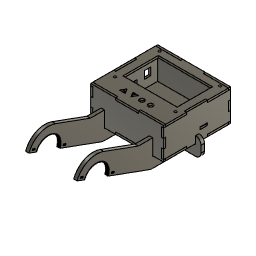
console (Autodesk Fusion 360 design; units mm, degrees)
Autodesk Fusion 360 part; units mm, degrees
sketch "Sketch2" plane through (0, 0, 0) normal (0, 0, 1) x (1, 0, 0)
  line L0 (-39.35, 25.65) -> (39.35, 25.65)
  line L1 (39.35, 25.65) -> (39.35, -25.65)
  line L2 (39.35, -25.65) -> (-39.35, -25.65)
  line L3 (-39.35, -25.65) -> (-39.35, 25.65)
  line L4 (-39.35, 25.65) -> (39.35, -25.65) construction
  line L5 (49.65, 35.65) -> (-50.35, 35.65)
  line L6 (-50.35, 35.65) -> (-50.35, -55.65)
  line L7 (-50.35, -55.65) -> (49.65, -55.65)
  line L8 (49.65, -55.65) -> (49.65, 35.65)
  line L9 (0, 35.516) -> (0, -32.6985) construction
  line L10 (-53.35, -58.65) -> (52.65, -58.65)
  line L11 (52.65, -58.65) -> (52.65, 38.65)
  line L12 (52.65, 38.65) -> (-53.35, 38.65)
  line L13 (-53.35, 38.65) -> (-53.35, -58.65)
  line L14 (-50.35, -55.65) -> (-53.35, -55.65)
  line L15 (-53.35, -25.2167) -> (-50.35, -25.2167)
  line L16 (-50.35, 5.2167) -> (-53.35, 5.2167)
  line L17 (-50.35, 35.65) -> (-53.35, 35.65)
  line L18 (-50.35, 35.65) -> (-50.35, 38.65)
  line L19 (-17.0167, 35.65) -> (-17.0167, 38.65)
  line L20 (16.3167, 35.65) -> (16.3167, 38.65)
  line L21 (49.65, 35.65) -> (49.65, 38.65)
  line L22 (49.65, 35.65) -> (52.65, 35.65)
  line L23 (49.65, 5.2167) -> (52.65, 5.2167)
  line L24 (49.65, -55.65) -> (52.65, -55.65)
  line L25 (49.65, -55.65) -> (49.65, -58.65)
  line L26 (16.3167, -55.65) -> (16.3167, -58.65)
  line L27 (-17.0167, -55.65) -> (-17.0167, -58.65)
  line L28 (-50.35, -55.65) -> (-50.35, -58.65)
  line L29 (-50.35, 37.15) -> (-17.0167, 37.15) construction
  line L30 (-17.0167, 37.15) -> (16.3167, 37.15) construction
  line L31 (16.3167, 37.15) -> (49.65, 37.15) construction
  line L32 (-51.85, 35.65) -> (-51.85, 5.2167) construction
  line L33 (-51.85, 5.2167) -> (-51.85, -25.2167) construction
  line L34 (-51.85, -25.2167) -> (-51.85, -55.65) construction
  line L35 (-50.35, -57.15) -> (-17.0167, -57.15) construction
  line L36 (-17.0167, -57.15) -> (16.3167, -57.15) construction
  line L37 (16.3167, -57.15) -> (49.65, -57.15) construction
  line L38 (49.65, -25.2167) -> (52.65, -25.2167)
  line L39 (51.15, -55.65) -> (51.15, -25.2167) construction
  line L40 (51.15, -25.2167) -> (51.15, 5.2167) construction
  line L41 (51.15, 5.2167) -> (51.15, 35.65) construction
  dimension "d1" = 78.7
  dimension "d2" = 51.3
  dimension "d3" = 100
  dimension "d4" = 10
  dimension "d6" = 30
  dimension "d16" = 3
  dimension "d113" = 11
  constraint horizontal L0
  constraint vertical L1
  constraint horizontal L2
  constraint vertical L3
  constraint midpoint origin L4
  constraint horizontal L5
  constraint vertical L6
  constraint horizontal L7
  constraint vertical L8
  constraint coincident origin L9
  constraint vertical L9
  constraint coincident L13 L14.end
  constraint perpendicular L13 L14
  constraint coincident L13 L15.start
  constraint coincident L6 L15.end
  constraint perpendicular L6 L15
  constraint coincident L6 L16.start
  constraint coincident L13 L16.end
  constraint perpendicular L13 L16
  constraint coincident L13 L17.end
  constraint perpendicular L13 L17
  constraint coincident L12 L18.end
  constraint perpendicular L12 L18
  constraint coincident L5 L19.start
  constraint coincident L12 L19.end
  constraint perpendicular L12 L19
  constraint coincident L5 L20.start
  constraint coincident L12 L20.end
  constraint perpendicular L12 L20
  constraint coincident L12 L21.end
  constraint perpendicular L12 L21
  constraint coincident L11 L22.end
  constraint perpendicular L11 L22
  constraint coincident L8 L23.start
  constraint coincident L11 L23.end
  constraint perpendicular L11 L23
  constraint coincident L11 L24.end
  constraint perpendicular L11 L24
  constraint coincident L10 L25.end
  constraint perpendicular L10 L25
  constraint coincident L7 L26.start
  constraint coincident L10 L26.end
  constraint perpendicular L10 L26
  constraint coincident L7 L27.start
  constraint coincident L10 L27.end
  constraint perpendicular L10 L27
  constraint coincident L10 L28.end
  constraint perpendicular L10 L28
  constraint midpoint L18 L29.start
  constraint midpoint L19 L29.end
  constraint midpoint L20 L30.end
  constraint midpoint L21 L31.end
  constraint equal L30 L31
  constraint equal L29 L30
  constraint midpoint L17 L32.start
  constraint midpoint L16 L32.end
  constraint midpoint L15 L33.end
  constraint midpoint L14 L34.end
  constraint equal L33 L34
  constraint equal L32 L34
  constraint midpoint L28 L35.start
  constraint midpoint L27 L35.end
  constraint midpoint L26 L36.end
  constraint midpoint L25 L37.end
  constraint equal L36 L37
  constraint equal L35 L36
  constraint coincident L8 L38.start
  constraint coincident L11 L38.end
  constraint perpendicular L11 L38
  constraint midpoint L24 L39.start
  constraint midpoint L38 L39.end
  constraint midpoint L23 L40.end
  constraint perpendicular L23 L41
  constraint midpoint L22 L41.end
  constraint equal L40 L41
  constraint equal L39 L40
  measures "d1" distance of L0.start L0.end
  measures "d2" distance of L0.end L1.end
  measures "d3" distance of L5.start L5.end
  measures "d4" distance of L0 L5
  measures "d6" distance of L2 L7
  measures "d113" distance of L3 L6
extrude "Extrude1" add sketch "Sketch2" along normal blind 3 contours L5 L6 L7 L8 | L8 L11 L22 L23 | L5 L12 L19 L20 | L8 L11 L24 L38 | L6 L13 L16 L17 | L7 L10 L26 L27 | L6 L13 L14 L15 makes body 1
sketch "Sketch3" plane through (0, 0, 0) normal (0, 0, -1) x (1, 0, 0)
  line L0 (-39.35, 25.65) -> (39.35, 25.65)
  line L1 (39.35, 25.65) -> (39.35, -25.65)
  line L2 (39.35, -25.65) -> (-39.35, -25.65)
  line L3 (-39.35, -25.65) -> (-39.35, 25.65)
  line L4 (-43.9, 32.65) -> (43.9, 32.65) construction
  line L5 (43.9, 32.65) -> (43.9, -32.15) construction
  line L6 (43.9, -32.15) -> (-43.9, -32.15) construction
  line L7 (-43.9, -32.15) -> (-43.9, 32.65) construction
  line L8 (-43.9, 32.65) -> (43.9, -32.15) construction
  circle A0 centre (-43.9, -32.15) radius 4
  circle A1 centre (43.9, -32.15) radius 4
  circle A2 centre (43.9, 32.65) radius 4
  circle A3 centre (-43.9, 32.65) radius 4
  circle A4 centre (-43.9, 32.65) radius 1.75
  circle A5 centre (43.9, 32.65) radius 1.75
  circle A6 centre (43.9, -32.15) radius 1.75
  circle A7 centre (-43.9, -32.15) radius 1.75
  line L9 (-53.35, 55.65) -> (-53.35, 25.2167)
  line L10 (-17.0167, -38.65) -> (16.3167, -38.65)
  line L11 (52.65, 25.2167) -> (52.65, 55.65)
  line L12 (16.3167, 58.65) -> (-17.0167, 58.65)
  line L13 (52.65, -5.2167) -> (49.65, -5.2167)
  line L14 (49.65, -5.2167) -> (49.65, 25.2167)
  line L15 (49.65, 25.2167) -> (52.65, 25.2167)
  line L16 (52.65, 55.65) -> (16.3167, 55.65)
  line L17 (16.3167, 55.65) -> (16.3167, 58.65)
  line L18 (-17.0167, 58.65) -> (-17.0167, 55.65)
  line L19 (-17.0167, 55.65) -> (-53.35, 55.65)
  line L20 (-53.35, 25.2167) -> (-50.35, 25.2167)
  line L21 (-50.35, 25.2167) -> (-50.35, -5.2167)
  line L22 (-50.35, -5.2167) -> (-53.35, -5.2167)
  line L23 (-53.35, -5.2167) -> (-53.35, -35.65)
  line L24 (-53.35, -35.65) -> (-17.0167, -35.65)
  line L25 (-17.0167, -35.65) -> (-17.0167, -38.65)
  line L26 (16.3167, -38.65) -> (16.3167, -35.65)
  line L27 (16.3167, -35.65) -> (52.65, -35.65)
  line L28 (52.65, -35.65) -> (52.65, -5.2167)
  line L29 (49.65, 55.65) -> (49.65, -35.65)
  line L30 (-17.0167, -35.65) -> (-53.35, -35.65)
  line L31 (0, 0) -> (0, 0.25) construction
  dimension "d9" = 87.8
  dimension "d10" = 64.8
  dimension "d11" = 8
  dimension "d12" = 3.5
  dimension "d55" = 3.5
  constraint horizontal L4
  constraint vertical L5
  constraint horizontal L6
  constraint vertical L7
  constraint coincident L6.end L7.start
  constraint coincident L5.end L6.start
  constraint coincident L4.end L5.start
  constraint coincident L4.start L7.end
  constraint equal A2 A3
  constraint equal A0 A3
  constraint equal A0 A1
  constraint concentric A3 A4
  constraint concentric A2 A5
  constraint concentric A1 A6
  constraint equal A6 A7
  constraint equal A4 A7
  constraint equal A4 A5
  constraint coincident L16 L29.start
  constraint coincident L27 L29.end
  constraint vertical L29
  constraint collinear L14 L29
  constraint coincident L31.start origin
  constraint midpoint L8 L31.end
  constraint vertical L31
  measures "d9" distance of L4.start L4.end
  measures "d10" distance of L4.end L5.end
  measures "d11" diameter of A1
  measures "d12" diameter of A4
  measures "d55" distance of L6 L30
extrude "Extrude2" add sketch "Sketch3" along normal blind 3 separate body contours A0 L24 L30 | A1 L27 | A2 | A3 picked at (-43.8564, -35.065) picked at (43.4291, -35.7307) makes body 2 at (47.895, -32.4506, -2) makes body 3 at (45.6659, 35.7391, -2) makes body 4 at (-39.905, -32.4506, -2) makes body 5 at (-42.3772, 28.4512, -1)
sketch "Sketch5" plane through (-50.35, 0, 0) normal (-1, 0, 0) x (0, -1, 0)
  line L0 (-5.2167, 0) -> (25.2167, 0)
  line L1 (25.2167, 0) -> (25.2167, 3)
  line L2 (25.2167, 3) -> (-5.2167, 3)
  line L3 (-5.2167, 3) -> (-5.2167, 0)
  line L4 (-38.65, 0) -> (-35.65, 0)
  line L5 (-35.65, 0) -> (-35.65, 3)
  line L6 (-35.65, 3) -> (-38.65, 3)
  line L7 (-38.65, 3) -> (-38.65, 0)
  line L8 (-35.65, 0) -> (-5.2167, 0)
  line L9 (-5.2167, 0) -> (-5.2167, 3)
  line L10 (-5.2167, 3) -> (-35.65, 3)
  line L11 (-35.65, 3) -> (-35.65, 0)
  line L12 (25.2167, 0) -> (55.65, 0)
  line L13 (55.65, 0) -> (55.65, 3)
  line L14 (55.65, 3) -> (25.2167, 3)
  line L15 (25.2167, 3) -> (25.2167, 0)
  line L16 (55.65, 0) -> (58.65, 0)
  line L17 (58.65, 0) -> (58.65, 3)
  line L18 (58.65, 3) -> (55.65, 3)
  line L19 (55.65, 3) -> (55.65, 0)
  line L20 (-35.65, 0) -> (55.65, 0)
  line L21 (55.65, 0) -> (55.65, -40)
  line L22 (55.65, -40) -> (-35.65, -40)
  line L23 (-35.65, -40) -> (-35.65, 0)
  line L24 (25.2167, 0) -> (55.65, 0)
  line L25 (-38.65, 0) -> (-35.65, 0)
  line L26 (-35.65, 0) -> (-35.65, -13.3333)
  line L27 (-35.65, -13.3333) -> (-38.65, -13.3333)
  line L28 (-38.65, -13.3333) -> (-38.65, 0)
  line L29 (-35.65, -40) -> (-38.65, -40)
  line L30 (-38.65, -40) -> (-38.65, -26.6667)
  line L31 (-38.65, -26.6667) -> (-35.65, -26.6667)
  line L32 (-35.65, -26.6667) -> (-35.65, -40)
  line L33 (-38.65, -13.3333) -> (-38.65, -26.6667) construction
  line L34 (55.65, 0) -> (58.65, 0)
  line L35 (58.65, 0) -> (58.65, -13.3333)
  line L36 (58.65, -13.3333) -> (55.65, -13.3333)
  line L37 (55.65, -13.3333) -> (55.65, 0)
  line L38 (55.65, -40) -> (58.65, -40)
  line L39 (58.65, -40) -> (58.65, -26.6667)
  line L40 (58.65, -26.6667) -> (55.65, -26.6667)
  line L41 (55.65, -26.6667) -> (55.65, -40)
  line L42 (58.65, -13.3333) -> (58.65, -26.6667) construction
  line L43 (-5.2167, -40) -> (25.2167, -40)
  line L44 (25.2167, -40) -> (25.2167, -43)
  line L45 (25.2167, -43) -> (-5.2167, -43)
  line L46 (-5.2167, -43) -> (-5.2167, -40)
  dimension "d31" = 40
  constraint horizontal L20
  constraint vertical L21
  constraint horizontal L22
  constraint vertical L23
  constraint coincident L4.end L5.start
  constraint coincident L12.end L13.start
  constraint horizontal L25
  constraint vertical L26
  constraint horizontal L27
  constraint vertical L28
  constraint coincident L23 L26.end
  constraint coincident L4.start L7.end
  constraint horizontal L29
  constraint vertical L30
  constraint horizontal L31
  constraint vertical L32
  constraint perpendicular L31 L33
  constraint equal L28 L33
  constraint equal L28 L30
  constraint horizontal L34
  constraint vertical L35
  constraint horizontal L36
  constraint vertical L37
  constraint coincident L16.end L17.start
  constraint horizontal L38
  constraint vertical L39
  constraint horizontal L40
  constraint vertical L41
  constraint collinear L35 L39
  constraint equal L35 L42
  constraint equal L35 L39
  constraint horizontal L43
  constraint vertical L44
  constraint horizontal L45
  constraint vertical L46
  constraint coincident L22 L43.start
  constraint equal L1 L44
  constraint equal L2 L45
  constraint collinear L3 L46
  measures "d31" distance of L22 L24
extrude "Extrude6" add sketch "Sketch5" along normal blind 3 separate body contours L0 L1 L2 L3 L9 L15 L20 | L0 L8 L12 L20 L21 L22 L23 L24 L26 L32 L37 L41 L43 | L4 L23 L25 L26 L27 L28 | L16 L21 L34 L35 L36 L37 | L23 L29 L30 L31 L32 | L21 L38 L39 L40 L41 | L22 L43 L44 L45 L46 makes body 6
sketch "Sketch4" plane through (-53.35, 0, 0) normal (-1, 0, 0) x (0, -1, 0)
  line L0 (25.2167, 0) -> (55.65, 0)
  line L1 (55.65, 0) -> (55.65, 3)
  line L2 (55.65, 3) -> (25.2167, 3)
  line L3 (25.2167, 3) -> (25.2167, 0)
  line L4 (-35.65, 0) -> (-5.2167, 0)
  line L5 (-5.2167, 0) -> (-5.2167, 3)
  line L6 (-5.2167, 3) -> (-35.65, 3)
  line L7 (-35.65, 3) -> (-35.65, 0)
  line L8 (-25.65, -17) -> (-16.65, -17)
  line L9 (-16.65, -17) -> (-16.65, -28)
  line L10 (-16.65, -28) -> (-25.65, -28)
  line L11 (-25.65, -28) -> (-25.65, -17)
  line L12 (-25.65, 3) -> (-25.65, -17) construction
  line L13 (-5.65, -31) -> (6.35, -31)
  line L14 (6.35, -31) -> (6.35, -23)
  line L15 (6.35, -23) -> (-5.65, -23)
  line L16 (-5.65, -23) -> (-5.65, -31)
  line L17 (-5.65, -23) -> (6.35, -31) construction
  point P0 (-25.65, 3)
  point P1 (25.65, 3)
  point P2 (0.35, -27)
  dimension "d114" = 17
  dimension "d115" = 11
  dimension "d116" = 9
  dimension "d118" = 17
  dimension "d119" = 12
  dimension "d120" = 8
  dimension "d125" = 1
  constraint horizontal L8
  constraint vertical L9
  constraint horizontal L10
  constraint vertical L11
  constraint coincident P0 L12.start
  constraint vertical L12
  constraint horizontal L13
  constraint vertical L14
  constraint horizontal L15
  constraint vertical L16
  constraint midpoint L17 P2
  measures "d114" distance of L4 L8
  measures "d115" distance of L8.end L9.end
  measures "d116" distance of L9.end L10.end
  measures "d118" distance of L9 P2
  measures "d119" distance of L14.end L15.end
  measures "d120" distance of L13.end L14.end
  measures "d125" distance of L10 P2
extrude "Extrude7" cut sketch "Sketch4" against normal through all contours L8 L9 L10 L11 | L13 L14 L15 L16 bodies 6
extrude "Extrude8" cut sketch "Sketch3" against normal through all contours A4 | A5 | A6 | A7 bodies 1
sketch "Sketch6" plane through (49.65, 0, 0) normal (1, 0, 0) x (0, 1, 0)
  line L0 (-58.65, -40) -> (-25.2167, -40)
  line L1 (-25.2167, -40) -> (-25.2167, -43)
  line L2 (-25.2167, -43) -> (5.2167, -43)
  line L3 (5.2167, -43) -> (5.2167, -40)
  line L4 (5.2167, -40) -> (38.65, -40)
  line L5 (38.65, -40) -> (38.65, -26.6667)
  line L6 (38.65, -26.6667) -> (35.65, -26.6667)
  line L7 (35.65, -26.6667) -> (35.65, -13.3333)
  line L8 (35.65, -13.3333) -> (38.65, -13.3333)
  line L9 (38.65, -13.3333) -> (38.65, 0)
  line L10 (38.65, 0) -> (5.2167, 0)
  line L11 (5.2167, 0) -> (5.2167, 3)
  line L12 (5.2167, 3) -> (-25.2167, 3)
  line L13 (-25.2167, 3) -> (-25.2167, 0)
  line L14 (-25.2167, 0) -> (-58.65, 0)
  line L15 (-58.65, 0) -> (-58.65, -13.3333)
  line L16 (-58.65, -13.3333) -> (-55.65, -13.3333)
  line L17 (-55.65, -13.3333) -> (-55.65, -26.6667)
  line L18 (-55.65, -26.6667) -> (-58.65, -26.6667)
  line L19 (-58.65, -26.6667) -> (-58.65, -40)
  line L20 (-6.35, -23) -> (5.65, -23)
  line L21 (5.65, -23) -> (5.65, -31)
  line L22 (5.65, -31) -> (-6.35, -31)
  line L23 (-6.35, -31) -> (-6.35, -23)
  line L24 (25.65, -17) -> (25.65, -28)
  line L25 (25.65, -28) -> (16.65, -28)
  line L26 (16.65, -28) -> (16.65, -17)
  line L27 (16.65, -17) -> (25.65, -17)
extrude "Extrude9" add sketch "Sketch6" along normal blind 3 separate body contours L0 L1 L2 L3 L4 L5 L6 L7 L8 L9 L10 L11 L12 L13 L14 L15 L16 L17 L18 L19 | L20 L21 L22 L23 | L24 L25 L26 L27 makes body 7
sketch "Sketch7" plane through (52.65, 0, 0) normal (1, 0, 0) x (0, 1, 0)
  line L0 (-58.65, -26.6667) -> (-58.65, -40)
  line L1 (-58.65, -40) -> (-25.2167, -40)
  line L2 (-25.2167, -40) -> (-25.2167, -43)
  line L3 (-25.2167, -43) -> (5.2167, -43)
  line L4 (5.2167, -43) -> (5.2167, -40)
  line L5 (5.2167, -40) -> (38.65, -40)
  line L6 (38.65, -40) -> (38.65, -26.6667)
  line L7 (38.65, -26.6667) -> (35.65, -26.6667)
  line L8 (35.65, -26.6667) -> (35.65, -13.3333)
  line L9 (35.65, -13.3333) -> (38.65, -13.3333)
  line L10 (38.65, -13.3333) -> (38.65, 0)
  line L11 (38.65, 0) -> (5.2167, 0)
  line L12 (5.2167, 0) -> (5.2167, 3)
  line L13 (5.2167, 3) -> (-25.2167, 3)
  line L14 (-25.2167, 3) -> (-25.2167, 0)
  line L15 (-25.2167, 0) -> (-58.65, 0)
  line L16 (-58.65, 0) -> (-58.65, -13.3333)
  line L17 (-58.65, -13.3333) -> (-55.65, -13.3333)
  line L18 (-55.65, -13.3333) -> (-55.65, -26.6667)
  line L19 (-55.65, -26.6667) -> (-58.65, -26.6667)
  line L20 (-5.6, -25.25) -> (4.9, -25.25)
  line L21 (4.9, -25.25) -> (4.9, -28.75)
  line L22 (4.9, -28.75) -> (-5.6, -28.75)
  line L23 (-5.6, -28.75) -> (-5.6, -25.25)
  line L24 (-6.35, -23) -> (5.65, -23)
  line L25 (5.65, -23) -> (5.65, -31)
  line L26 (5.65, -31) -> (-6.35, -31)
  line L27 (-6.35, -31) -> (-6.35, -23)
  line L28 (-5.6, -25.25) -> (4.9, -28.75) construction
  line L29 (5.65, -31) -> (-6.35, -23) construction
  dimension "d122" = 10.5
  dimension "d123" = 3.5
  constraint horizontal L20
  constraint vertical L21
  constraint horizontal L22
  constraint vertical L23
  constraint coincident L25.end L26.start
  constraint coincident L24.start L27.end
  constraint midpoint L28 L29
  measures "d122" distance of L20.start L20.end
  measures "d123" distance of L20.end L21.end
extrude "Extrude10" cut sketch "Sketch7" against normal through all contours L20 L21 L22 L23 bodies 7
sketch "Sketch8" plane through (0, -55.65, 0) normal (0, -1, 0) x (1, 0, 0)
  line L0 (-53.35, 0) -> (-17.0167, 0)
  line L1 (-17.0167, 0) -> (-17.0167, 3)
  line L2 (-17.0167, 3) -> (-53.35, 3)
  line L3 (-53.35, 3) -> (-53.35, 0)
  line L4 (-17.0167, 0) -> (16.3167, 0)
  line L5 (16.3167, 0) -> (16.3167, 3)
  line L6 (16.3167, 3) -> (-17.0167, 3)
  line L7 (-17.0167, 3) -> (-17.0167, 0)
  line L8 (16.3167, 0) -> (52.65, 0)
  line L9 (52.65, 0) -> (52.65, 3)
  line L10 (52.65, 3) -> (16.3167, 3)
  line L11 (16.3167, 3) -> (16.3167, 0)
  line L12 (49.65, 0) -> (49.65, -13.3333)
  line L13 (49.65, -13.3333) -> (52.65, -13.3333)
  line L14 (52.65, -13.3333) -> (52.65, 0)
  line L15 (52.65, 0) -> (49.65, 0)
  line L16 (49.65, -13.3333) -> (49.65, -26.6667)
  line L17 (49.65, -26.6667) -> (52.65, -26.6667)
  line L18 (52.65, -26.6667) -> (52.65, -13.3333)
  line L19 (52.65, -13.3333) -> (49.65, -13.3333)
  line L20 (49.65, -26.6667) -> (49.65, -40)
  line L21 (49.65, -40) -> (52.65, -40)
  line L22 (52.65, -40) -> (52.65, -26.6667)
  line L23 (52.65, -26.6667) -> (49.65, -26.6667)
  line L24 (-50.35, -40) -> (-50.35, -26.6667)
  line L25 (-50.35, -26.6667) -> (-53.35, -26.6667)
  line L26 (-53.35, -26.6667) -> (-53.35, -40)
  line L27 (-53.35, -40) -> (-50.35, -40)
  line L28 (-50.35, -13.3333) -> (-50.35, 0)
  line L29 (-50.35, 0) -> (-53.35, 0)
  line L30 (-53.35, 0) -> (-53.35, -13.3333)
  line L31 (-53.35, -13.3333) -> (-50.35, -13.3333)
  line L32 (-50.35, -26.6667) -> (-50.35, -13.3333)
  line L33 (-50.35, -13.3333) -> (-53.35, -13.3333)
  line L34 (-53.35, -13.3333) -> (-53.35, -26.6667)
  line L35 (-53.35, -26.6667) -> (-50.35, -26.6667)
  line L36 (-50.35, -40) -> (49.65, -40)
  line L37 (-53.35, -40) -> (-17.0167, -40)
  line L38 (-17.0167, -40) -> (-17.0167, -43)
  line L39 (-17.0167, -43) -> (-53.35, -43)
  line L40 (-53.35, -43) -> (-53.35, -40)
  line L41 (-17.0167, -43) -> (16.3167, -43)
  line L42 (16.3167, -43) -> (16.3167, -40)
  line L43 (16.3167, -40) -> (-17.0167, -40)
  line L44 (-17.0167, -40) -> (-17.0167, -43)
  line L45 (16.3167, -43) -> (52.65, -43)
  line L46 (52.65, -43) -> (52.65, -40)
  line L47 (52.65, -40) -> (16.3167, -40)
  line L48 (16.3167, -40) -> (16.3167, -43)
  constraint coincident L24.start L27.end
  constraint coincident L20.end L21.start
  constraint horizontal L37
  constraint vertical L38
  constraint horizontal L39
  constraint vertical L40
  constraint coincident L26.end L27.start
  constraint horizontal L41
  constraint vertical L42
  constraint horizontal L43
  constraint vertical L44
  constraint coincident L36 L42.end
  constraint horizontal L45
  constraint vertical L46
  constraint horizontal L47
  constraint vertical L48
  constraint coincident L21.end L22.start
  constraint collinear L11 L48
  constraint collinear L1 L38
  constraint equal L1 L38
extrude "Extrude11" add sketch "Sketch8" along normal blind 3 separate body contours L0 L1 L2 L3 L7 L29 | L0 L4 L8 L12 L16 L20 L24 L28 L32 L36 L37 L43 L47 | L25 L31 L32 L33 L34 L35 | L5 L8 L9 L10 L11 L15 | L27 L36 L37 L38 L39 L40 L44 | L13 L16 L17 L18 L19 L23 | L21 L36 L42 L45 L46 L47 L48 makes body 8
sketch "Sketch9" plane through (0, 35.65, 0) normal (0, 1, 0) x (-1, 0, 0)
  line L0 (-52.65, 0) -> (-16.3167, 0)
  line L1 (-16.3167, 0) -> (-16.3167, 3)
  line L2 (-16.3167, 3) -> (-52.65, 3)
  line L3 (-52.65, 3) -> (-52.65, 0)
  line L4 (-16.3167, -40) -> (17.0167, -40)
  line L5 (17.0167, -40) -> (17.0167, -43)
  line L6 (17.0167, -43) -> (53.35, -43)
  line L7 (53.35, -43) -> (53.35, -40)
  line L8 (53.35, -40) -> (50.35, -40)
  line L9 (50.35, -40) -> (50.35, -26.6667)
  line L10 (50.35, -26.6667) -> (53.35, -26.6667)
  line L11 (53.35, -26.6667) -> (53.35, -13.3333)
  line L12 (53.35, -13.3333) -> (50.35, -13.3333)
  line L13 (50.35, -13.3333) -> (50.35, 0)
  line L14 (50.35, 0) -> (53.35, 0)
  line L15 (53.35, 0) -> (53.35, 3)
  line L16 (53.35, 3) -> (17.0167, 3)
  line L17 (17.0167, 3) -> (17.0167, 0)
  line L18 (17.0167, 0) -> (-16.3167, 0)
  line L19 (-16.3167, 0) -> (-16.3167, 3)
  line L20 (-16.3167, 3) -> (-52.65, 3)
  line L21 (-52.65, 3) -> (-52.65, 0)
  line L22 (-52.65, 0) -> (-49.65, 0)
  line L23 (-49.65, 0) -> (-49.65, -13.3333)
  line L24 (-49.65, -13.3333) -> (-52.65, -13.3333)
  line L25 (-52.65, -13.3333) -> (-52.65, -26.6667)
  line L26 (-52.65, -26.6667) -> (-49.65, -26.6667)
  line L27 (-49.65, -26.6667) -> (-49.65, -40)
  line L28 (-49.65, -40) -> (-52.65, -40)
  line L29 (-52.65, -40) -> (-52.65, -43)
  line L30 (-52.65, -43) -> (-16.3167, -43)
  line L31 (-16.3167, -43) -> (-16.3167, -40)
extrude "Extrude12" add sketch "Sketch9" along normal blind 3 separate body makes body 9
sketch "Sketch10" plane through (0, 0, -40) normal (0, 0, -1) x (1, 0, 0)
  line L0 (52.65, -5.2167) -> (49.65, -5.2167)
  line L1 (49.65, -5.2167) -> (49.65, 25.2167)
  line L2 (49.65, 25.2167) -> (52.65, 25.2167)
  line L3 (52.65, 25.2167) -> (52.65, 55.65)
  line L4 (52.65, 55.65) -> (16.3167, 55.65)
  line L5 (16.3167, 55.65) -> (16.3167, 58.65)
  line L6 (16.3167, 58.65) -> (-17.0167, 58.65)
  line L7 (-17.0167, 58.65) -> (-17.0167, 55.65)
  line L8 (-17.0167, 55.65) -> (-53.35, 55.65)
  line L9 (-53.35, 55.65) -> (-53.35, 25.2167)
  line L10 (-53.35, 25.2167) -> (-50.35, 25.2167)
  line L11 (-50.35, 25.2167) -> (-50.35, -5.2167)
  line L12 (-50.35, -5.2167) -> (-53.35, -5.2167)
  line L13 (-53.35, -5.2167) -> (-53.35, -35.65)
  line L14 (-53.35, -35.65) -> (-17.0167, -35.65)
  line L15 (-17.0167, -35.65) -> (-17.0167, -38.65)
  line L16 (-17.0167, -38.65) -> (16.3167, -38.65)
  line L17 (16.3167, -38.65) -> (16.3167, -35.65)
  line L18 (16.3167, -35.65) -> (52.65, -35.65)
  line L19 (52.65, -35.65) -> (52.65, -5.2167)
extrude "Extrude13" add sketch "Sketch10" along normal blind 3 separate body makes body 10
sketch "Sketch11" plane through (0, 0, 3) normal (0, 0, 1) x (-1, 0, 0)
  circle A0 centre (-43.9, 32.65) radius 1.75
  circle A1 centre (-43.9, -32.15) radius 1.75
  circle A2 centre (43.9, 32.65) radius 1.75
  circle A3 centre (43.9, -32.15) radius 1.75
  line L0 (-39.35, 25.65) -> (39.35, 25.65)
  line L1 (39.35, 25.65) -> (39.35, -25.65)
  line L2 (39.35, -25.65) -> (-39.35, -25.65)
  line L3 (-39.35, -25.65) -> (-39.35, 25.65)
  line L4 (-49.65, -5.2167) -> (-52.65, -5.2167)
  line L5 (-52.65, -5.2167) -> (-52.65, -35.65)
  line L6 (-52.65, -35.65) -> (-16.3167, -35.65)
  line L7 (-16.3167, -35.65) -> (-16.3167, -38.65)
  line L8 (-16.3167, -38.65) -> (17.0167, -38.65)
  line L9 (17.0167, -38.65) -> (17.0167, -35.65)
  line L10 (17.0167, -35.65) -> (53.35, -35.65)
  line L11 (53.35, -35.65) -> (53.35, -5.2167)
  line L12 (53.35, -5.2167) -> (50.35, -5.2167)
  line L13 (50.35, -5.2167) -> (50.35, 25.2167)
  line L14 (50.35, 25.2167) -> (53.35, 25.2167)
  line L15 (53.35, 25.2167) -> (53.35, 55.65)
  line L16 (53.35, 55.65) -> (17.0167, 55.65)
  line L17 (17.0167, 55.65) -> (17.0167, 58.65)
  line L18 (17.0167, 58.65) -> (-16.3167, 58.65)
  line L19 (-16.3167, 58.65) -> (-16.3167, 55.65)
  line L20 (-16.3167, 55.65) -> (-52.65, 55.65)
  line L21 (-52.65, 55.65) -> (-52.65, 25.2167)
  line L22 (-52.65, 25.2167) -> (-49.65, 25.2167)
  line L23 (-49.65, 25.2167) -> (-49.65, -5.2167)
  line L24 (50.35, 25.2167) -> (50.35, 55.65)
  line L25 (50.35, 35.65) -> (-48.1566, 35.65)
  line L26 (-49.65, 25.2167) -> (-49.65, 55.65)
  line L27 (19.8467, 42.65) -> (7.3467, 42.65) construction
  line L28 (7.3467, 42.65) -> (-5.1533, 42.65) construction
  line L29 (-5.1533, 42.65) -> (-17.6533, 42.65) construction
  line L30 (1.0967, 42.65) -> (1.0967, 35.65) construction
  line L31 (17.0167, 55.65) -> (-16.3167, 55.65) construction
  line L32 (23.8467, 46.1141) -> (15.8467, 46.1141)
  line L33 (15.8467, 46.1141) -> (19.8467, 39.1859)
  line L34 (19.8467, 39.1859) -> (23.8467, 46.1141)
  line L35 (11.3467, 39.1859) -> (3.3467, 39.1859)
  line L36 (3.3467, 39.1859) -> (7.3467, 46.1141)
  line L37 (7.3467, 46.1141) -> (11.3467, 39.1859)
  line L38 (7.3467, 39.1859) -> (7.3467, 46.1141) construction
  line L39 (19.8467, 39.1859) -> (19.8467, 46.1141) construction
  circle A4 centre (-5.1533, 42.65) radius 3.4641
  circle A5 centre (-17.6533, 42.65) radius 3.4641
  point P0 (19.8467, 42.65)
  point P1 (7.3467, 42.65)
  dimension "d50" = 10
  dimension "d51" = 12.5
  dimension "d52" = 8
  dimension "d54" = 7
  constraint coincident L13.end L14.start
  constraint coincident L16 L24.end
  constraint perpendicular L16 L24
  constraint coincident L24 L25.start
  constraint perpendicular L24 L25
  constraint coincident L22.end L23.start
  constraint coincident L20 L26.end
  constraint perpendicular L20 L26
  constraint horizontal L27
  constraint parallel L27 L28
  constraint parallel L28 L29
  constraint equal L28 L29
  constraint equal L27 L28
  constraint midpoint L28 L30.start
  constraint midpoint L25 L30.end
  constraint perpendicular L25 L30
  constraint coincident L16.end L17.start
  constraint coincident L19.end L20.start
  constraint perpendicular L1 L32
  constraint equal L32 L34
  constraint equal L32 L33
  constraint coincident L27 P0
  constraint coincident P0 L27.start
  constraint parallel L27 L35
  constraint equal L35 L37
  constraint equal L35 L36
  constraint equal L33 L37
  constraint midpoint L35 L38.start
  constraint coincident L38 P1
  constraint midpoint L38 P1
  constraint midpoint L32 L39.end
  constraint midpoint P0 L39
  constraint coincident P1 L27.end
  constraint coincident L28.end L29.start
  constraint coincident L29.end A5.centre
  constraint tangent L35 A4
  constraint equal A4 A5
  measures "d50" distance of L0 L25
  measures "d51" distance of P0 P1
  measures "d52" distance of L35.start L35.end
  measures "d54" distance of L30.start L30.end
extrude "Extrude14" cut sketch "Sketch11" against normal through all contours L32 L33 L34 | L35 L36 L37 | A4 | A5 bodies 1
sketch "Sketch14" plane through (0, 0, 3) normal (0, 0, 1) x (-1, 0, 0)
  line L0 (3.3467, 39.1859) -> (7.3467, 46.1141)
  line L1 (7.3467, 46.1141) -> (11.3467, 39.1859)
  line L2 (11.3467, 39.1859) -> (3.3467, 39.1859)
  circle A0 centre (-5.1533, 42.65) radius 3.4641
  line L3 (23.8467, 46.1141) -> (19.8467, 39.1859)
  line L4 (19.8467, 39.1859) -> (15.8467, 46.1141)
  line L5 (15.8467, 46.1141) -> (23.8467, 46.1141)
  circle A1 centre (-17.6533, 42.65) radius 3.4641
  circle A2 centre (-43.9, 32.65) radius 1.75
  circle A3 centre (-43.9, -32.15) radius 1.75
  circle A4 centre (43.9, 32.65) radius 1.75
  circle A5 centre (43.9, -32.15) radius 1.75
  line L6 (-39.35, 25.65) -> (39.35, 25.65)
  line L7 (39.35, 25.65) -> (39.35, -25.65)
  line L8 (39.35, -25.65) -> (-39.35, -25.65)
  line L9 (-39.35, -25.65) -> (-39.35, 25.65)
  line L10 (-49.65, -5.2167) -> (-52.65, -5.2167)
  line L11 (-52.65, -5.2167) -> (-52.65, -35.65)
  line L12 (-52.65, -35.65) -> (-16.3167, -35.65)
  line L13 (-16.3167, -35.65) -> (-16.3167, -38.65)
  line L14 (-16.3167, -38.65) -> (17.0167, -38.65)
  line L15 (17.0167, -38.65) -> (17.0167, -35.65)
  line L16 (17.0167, -35.65) -> (53.35, -35.65)
  line L17 (53.35, -35.65) -> (53.35, -5.2167)
  line L18 (53.35, -5.2167) -> (50.35, -5.2167)
  line L19 (50.35, -5.2167) -> (50.35, 25.2167)
  line L20 (50.35, 25.2167) -> (53.35, 25.2167)
  line L21 (53.35, 25.2167) -> (53.35, 55.65)
  line L22 (53.35, 55.65) -> (17.0167, 55.65)
  line L23 (17.0167, 55.65) -> (17.0167, 58.65)
  line L24 (17.0167, 58.65) -> (-16.3167, 58.65)
  line L25 (-16.3167, 58.65) -> (-16.3167, 55.65)
  line L26 (-16.3167, 55.65) -> (-52.65, 55.65)
  line L27 (-52.65, 55.65) -> (-52.65, 25.2167)
  line L28 (-52.65, 25.2167) -> (-49.65, 25.2167)
  line L29 (-49.65, 25.2167) -> (-49.65, -5.2167)
  circle A6 centre (-17.6533, 42.65) radius 3.1641
  circle A7 centre (-5.1533, 42.65) radius 3.1641
  line L30 (7.3467, 45.5141) -> (10.8271, 39.4859)
  line L31 (10.8271, 39.4859) -> (3.8663, 39.4859)
  line L32 (3.8663, 39.4859) -> (7.3467, 45.5141)
  line L33 (23.3271, 45.8141) -> (19.8467, 39.7859)
  line L34 (19.8467, 39.7859) -> (16.3663, 45.8141)
  line L35 (16.3663, 45.8141) -> (23.3271, 45.8141)
  line L36 (26.4448, 47.6141) -> (19.8467, 36.1859)
  line L37 (19.8467, 36.1859) -> (13.2486, 47.6141)
  line L38 (13.2486, 47.6141) -> (26.4448, 47.6141)
  line L39 (7.3467, 49.1141) -> (13.9448, 37.6859)
  line L40 (13.9448, 37.6859) -> (0.7486, 37.6859)
  line L41 (0.7486, 37.6859) -> (7.3467, 49.1141)
  circle A8 centre (-5.1533, 42.65) radius 4.9641
  circle A9 centre (-17.6533, 42.65) radius 4.9641
  line L42 (29.4429, 46.1141) -> (27.8654, 46.1141)
  line L43 (27.8654, 46.1141) -> (-27.5893, 46.1141)
  dimension "d59" = -0.3
  dimension "d60" = -0.3
  dimension "d61" = 0.3
  dimension "d62" = 0.3
  dimension "d63" = -1.5
  dimension "d64" = -1.5
  dimension "d65" = 1.5
  dimension "d66" = 1.5
  constraint parallel L35 L42
  constraint parallel L42 L43
  constraint collinear L5 L43
extrude "Extrude15" add sketch "Sketch14" against normal blind 4 from surface at 1 separate body contours A6 | A7 | L30 L31 L32 | L33 L34 L35 makes body 11 at (-8.5069, -43.5047, 2.6667) makes body 12 at (2.0049, -42.335, 1.3333) makes body 13 at (-18.6866, -41.7953, 2.6667) makes body 14 at (14.5049, -42.335, 1.3333)
extrude "Extrude16" add sketch "Sketch14" against normal blind 2 from surface at -3 contours L39 L40 L41 L43 | L0 L1 L2 | A0 | A8 L43 | L3 L4 L36 L37 L43 | L3 L4 L5 L43 | A1 | A9 L43 | A6 | A7 | L30 L31 L32 | L33 L34 L35 picked at (-8.5706, 45.5086) picked at (-21.0706, 45.5086) bodies 11 12 13 14
fillet "Fillet2" radius 1 4 faces at (-7.3467, -41.4953, 4) (5.9685, -41.8254, 4) (-19.8467, -43.8047, 4) (19.3399, -43.3348, 4) on bodies 11 12 13 14
ref_plane "WorkPlane3" through (-0.35, -10, -20) normal (1, 0, 0) x (0, 0, -1)
sketch "Sketch15" plane through (-0.35, 0, 0) normal (1, 0, 0) x (0, 1, 0)
  circle A0 centre (-140.6017, -29.7621) radius 17.75
  line L0 (38.5, 0) -> (38.5, -13.3333)
  line L1 (38.5, -26.6667) -> (38.5, -13.3333)
  line L2 (38.5, -26.6667) -> (38.5, -40)
  line L3 (38.5, -43) -> (38.5, -40)
  line L4 (35.5, -43) -> (38.5, -43)
  line L5 (5.1667, -43) -> (35.5, -43)
  line L6 (5.1667, -43) -> (-25.1667, -43)
  line L7 (-55.5, -43) -> (-25.1667, -43)
  line L8 (-55.5, -43) -> (-58.5, -43)
  line L9 (-58.5, -40) -> (-58.5, -43)
  line L10 (-58.5, -40) -> (-58.5, -26.6667)
  line L11 (-58.5, -13.3333) -> (-58.5, -26.6667)
  line L12 (-58.5, -13.3333) -> (-58.5, 0)
  line L13 (39, 0) -> (39, -13.3333)
  line L14 (39, -26.6667) -> (39, -13.3333)
  line L15 (39, -26.6667) -> (39, -40)
  line L16 (39, -43.5) -> (39, -40)
  line L17 (35.5, -43.5) -> (39, -43.5)
  line L18 (5.1667, -43.5) -> (35.5, -43.5)
  line L19 (5.1667, -43.5) -> (-25.1667, -43.5)
  line L20 (-55.5, -43.5) -> (-25.1667, -43.5)
  line L21 (-55.5, -43.5) -> (-59, -43.5)
  line L22 (-59, -40) -> (-59, -43.5)
  line L23 (-59, -40) -> (-59, -26.6667)
  line L24 (-59, -13.3333) -> (-59, -26.6667)
  arc A1 (54.0001, -35) -> (39, -20) centre (39, -35.0001) ccw
  line L25 (54.0001, -35) -> (54.0001, -43)
  line L26 (39, -20) -> (54.5526, -20) construction
  arc A2 (38.5465, -58.5) -> (54.0001, -43) centre (38.5, -43) ccw
  line L27 (-123.9221, -35.8329) -> (-140.6017, -29.7621) construction
  line L28 (-79.7087, -20) -> (-130.3411, -1.5713)
  arc A3 (-130.3411, -1.5713) -> (-168.7924, -19.5015) centre (-140.6017, -29.7621) ccw
  line L29 (-140.6017, -29.7621) -> (-157.2812, -23.6912) construction
  arc A4 (-64.1303, -57.5954) -> (-59, -58.5) centre (-59, -43.5) ccw
  line L30 (38.5465, -58.5) -> (-59, -58.5)
  line L31 (-64.1303, -57.5954) -> (-123.9221, -35.8329)
  line L32 (-157.2812, -23.6912) -> (-168.7924, -19.5015)
  line L33 (-160.7722, -19.7602) -> (-163.5913, -18.7341)
  line L34 (-163.8902, -18.0932) -> (-163.5481, -17.1535)
  line L35 (-162.9073, -16.8547) -> (-160.0882, -17.8808)
  line L36 (-159.7894, -18.5216) -> (-160.1314, -19.4613)
  line L37 (-59, -20) -> (-79.7087, -20)
  line L38 (-162.1818, -19.2471) -> (-163.0368, -21.5964) construction
  line L39 (-140.6017, -29.7621) -> (-135.301, -15.1987) construction
  line L40 (-115.2611, -35.7928) -> (-114.919, -34.8531)
  line L41 (-115.2179, -34.2122) -> (-118.037, -33.1862)
  line L42 (-118.721, -35.0656) -> (-115.9019, -36.0916)
  line L43 (-118.6778, -33.485) -> (-119.0198, -34.4247)
  line L44 (-7.7267, -58.5) -> (-12.7267, -58.5)
  line L45 (-12.7267, -58.5) -> (-12.7267, -51)
  line L46 (-12.7267, -51) -> (-7.7267, -51)
  line L47 (-7.7267, -51) -> (-7.7267, -58.5)
  line L48 (-10.2267, -58.5) -> (-10.2267, -43.5) construction
  arc A5 (-162.9073, -16.8547) -> (-163.5481, -17.1535) centre (-163.0783, -17.3246) ccw
  arc A6 (-163.8902, -18.0932) -> (-163.5913, -18.7341) centre (-163.4203, -18.2642) ccw
  arc A7 (-160.7722, -19.7602) -> (-160.1314, -19.4613) centre (-160.6012, -19.2903) ccw
  arc A8 (-159.7894, -18.5216) -> (-160.0882, -17.8808) centre (-160.2592, -18.3506) ccw
  arc A9 (-118.037, -33.1862) -> (-118.6778, -33.485) centre (-118.208, -33.656) ccw
  arc A10 (-119.0198, -34.4247) -> (-118.721, -35.0656) centre (-118.55, -34.5957) ccw
  arc A11 (-114.919, -34.8531) -> (-115.2179, -34.2122) centre (-115.3889, -34.6821) ccw
  arc A12 (-115.9019, -36.0916) -> (-115.2611, -35.7928) centre (-115.7309, -35.6218) ccw
  point P0 (-160.3024, -19.9312)
  point P1 (-164.0612, -18.5631)
  point P2 (-163.3771, -16.6837)
  dimension "d72" = 35.5
  dimension "d73" = 0.5
  dimension "d79" = 20
  dimension "d80" = 15
  dimension "d81" = 15
  dimension "d82" = 82.75
  dimension "d83" = 4
  dimension "d85" = 2
  dimension "d87" = 30
  dimension "d88" = 2.5
  dimension "d89" = 4.125
  dimension "d93" = 5
  dimension "d126" = 0.5
  constraint midpoint L14 A1.end
  constraint vertical L25
  constraint tangent A1 L25
  constraint perpendicular L14 L26
  constraint tangent A1 L26
  constraint coincident L25 A2.end
  constraint coincident L3.start L4.end
  constraint tangent L25 A2
  constraint coincident A0.centre L27.end
  constraint coincident A0 L27.start
  constraint coincident L28.end A3.start
  constraint tangent L28 A3
  constraint parallel L27 L29
  constraint coincident L21.end L22.end
  constraint tangent A4 L31
  constraint tangent A4 L30
  constraint parallel L28 L31
  constraint coincident A0 L29.end
  constraint parallel L27 L32
  constraint horizontal L30
  constraint collinear L27 L31
  constraint parallel L32 L33
  constraint perpendicular L32 L34
  constraint perpendicular L34 L35
  constraint parallel L34 L36
  constraint midpoint L24 L37.start
  constraint perpendicular L24 L37
  constraint coincident L28.start L37.end
  constraint midpoint L32 L38.end
  constraint perpendicular L32 L38
  constraint perpendicular L27 L39
  constraint horizontal L44
  constraint vertical L45
  constraint horizontal L46
  constraint vertical L47
  constraint midpoint L30 L44
  constraint midpoint L44 L48.start
  constraint coincident L19 L48.end
  constraint perpendicular L19 L48
  constraint midpoint L46 L48
  constraint coincident P2 L34
  constraint coincident P2 L35
  constraint tangent L34 A5
  constraint tangent L35 A5
  constraint coincident L33 L38.start
  constraint coincident P1 L33
  constraint coincident P1 L34
  constraint tangent L33 A6
  constraint tangent L34 A6
  constraint equal A5 A6
  constraint coincident P0 L33
  constraint coincident P0 L36
  constraint tangent L33 A7
  constraint tangent L36 A7
  constraint equal A5 A7
  constraint tangent L35 A8
  constraint tangent L36 A8
  constraint equal A5 A8
  constraint tangent L41 A9
  constraint tangent L43 A9
  constraint equal A5 A9
  constraint tangent L42 A10
  constraint tangent L43 A10
  constraint equal A5 A10
  constraint tangent L40 A11
  constraint tangent L41 A11
  constraint equal A5 A11
  constraint tangent L40 A12
  constraint tangent L42 A12
  constraint equal A5 A12
  measures "d72" diameter of A0
  measures "d79" angle of L30 L31
  measures "d80" distance of L19 L30
  measures "d81" distance of L15 L25
  measures "d82" distance of A0.centre L21.end
  measures "d83" distance of P0 P1
  measures "d85" distance of P1 P2
  measures "d87" distance of L28 L31
  measures "d88" distance of L38.start L38.end
  measures "d89" distance of L29.end L36
  measures "d93" distance of L45.end L46.end
  measures "d126" radius of A5
extrude "Extrude17" add sketch "Sketch15" along normal blind 5 from surface at 32.5 separate body contours A0 L14 L15 L16 L17 L18 L19 L20 L21 L22 L23 L24 A1 L25 A2 L28 A3 A4 L30 L31 L32 L37 L45 L46 L47 makes body 15
extrude "Extrude18" add sketch "Sketch15" against normal blind 5 from surface at -32.5 separate body contours A0 L14 L15 L16 L17 L18 L19 L20 L21 L22 L23 L24 A1 L25 A2 L28 A3 A4 L30 L31 L32 L37 L45 L46 L47 makes body 16
sketch "Sketch16" plane through (0, -12.7267, 0) normal (0, 1, 0) x (-1, 0, 0)
  line L0 (-52.65, -43) -> (-49.65, -43)
  line L1 (-49.65, -43) -> (-52.65, -43)
  line L2 (-52.65, -43) -> (-16.3167, -43)
  line L3 (-16.3167, -43) -> (17.0167, -43)
  line L4 (17.0167, -43) -> (53.35, -43)
  line L5 (53.35, -43) -> (50.35, -43)
  line L6 (50.35, -43) -> (53.35, -43)
  line L7 (53.35, -43) -> (17.0167, -43)
  line L8 (17.0167, -43) -> (-16.3167, -43)
  line L9 (-16.3167, -43) -> (-52.65, -43)
  line L10 (53.35, -40) -> (53.35, -26.6667)
  line L11 (53.35, -26.6667) -> (53.35, -13.3333)
  line L12 (53.35, -13.3333) -> (53.35, 0)
  line L13 (53.35, 0) -> (53.35, 3)
  line L14 (53.35, 3) -> (53.35, 0)
  line L15 (53.35, 0) -> (53.35, -13.3333)
  line L16 (53.35, -13.3333) -> (53.35, -26.6667)
  line L17 (53.35, -26.6667) -> (53.35, -40)
  line L18 (53.35, -40) -> (53.35, -43)
  line L19 (53.35, -43) -> (53.35, -40)
  line L20 (-52.65, -26.6667) -> (-52.65, -40)
  line L21 (-52.65, -40) -> (-52.65, -43)
  line L22 (-52.65, -43) -> (-52.65, -40)
  line L23 (-52.65, -40) -> (-52.65, -26.6667)
  line L24 (-52.65, -26.6667) -> (-52.65, -13.3333)
  line L25 (-52.65, -13.3333) -> (-52.65, 0)
  line L26 (-52.65, 0) -> (-52.65, 3)
  line L27 (-52.65, 3) -> (-52.65, 0)
  line L28 (-52.65, 0) -> (-52.65, -13.3333)
  line L29 (-52.65, -13.3333) -> (-52.65, -26.6667)
  line L30 (32.85, -51) -> (32.85, -58.5)
  line L31 (32.85, -58.5) -> (37.85, -58.5)
  line L32 (37.85, -58.5) -> (37.85, -51)
  line L33 (37.85, -51) -> (32.85, -51)
  line L34 (-32.15, -58.5) -> (-32.15, -51)
  line L35 (-32.15, -51) -> (-37.15, -51)
  line L36 (-37.15, -51) -> (-37.15, -58.5)
  line L37 (-37.15, -58.5) -> (-32.15, -58.5)
  line L38 (53.5, -32.4999) -> (58.2173, -32.4999) construction
  line L39 (37.85, -58.5) -> (53.85, -58.5)
  arc A0 (53.85, -58.5) -> (61.85, -50.5) centre (53.85, -50.5) ccw
  line L40 (61.85, -40.4999) -> (61.85, -50.5)
  line L41 (-53.15, -13.3333) -> (-53.15, -26.6667)
  line L42 (-53.15, -26.6667) -> (-53.15, -40)
  line L43 (-53.15, -43.5) -> (-53.15, -40)
  line L44 (-16.3167, -43.5) -> (-53.15, -43.5)
  line L45 (-16.3167, -43.5) -> (17.0167, -43.5)
  line L46 (53.85, -43.5) -> (17.0167, -43.5)
  line L47 (53.85, -40) -> (53.85, -43.5)
  line L48 (53.85, -40) -> (53.85, -26.6667)
  line L49 (53.85, -13.3333) -> (53.85, -26.6667)
  arc A1 (61.85, -40.4999) -> (53.85, -32.4999) centre (53.85, -40.4999) ccw
  line L50 (-32.15, -58.5) -> (32.85, -58.5)
  line L51 (32.85, -51) -> (37.85, -51)
  line L52 (37.85, -51) -> (37.85, -43.5)
  line L53 (37.85, -43.5) -> (32.85, -43.5)
  line L54 (32.85, -43.5) -> (32.85, -51)
  line L55 (-37.15, -51) -> (-32.15, -51)
  line L56 (-32.15, -51) -> (-32.15, -43.5)
  line L57 (-32.15, -43.5) -> (-37.15, -43.5)
  line L58 (-37.15, -43.5) -> (-37.15, -51)
  line L59 (0.35, -58.5) -> (0.35, -43.5)
  line L60 (-37.15, -58.5) -> (-53.15, -58.5)
  arc A2 (-61.15, -50.5) -> (-53.15, -58.5) centre (-53.15, -50.5) ccw
  line L61 (-61.15, -40.4999) -> (-61.15, -50.5)
  arc A3 (-53.15, -32.4999) -> (-61.15, -40.4999) centre (-53.15, -40.4999) ccw
  line L62 (53.35, -23) -> (53.35, -31)
  line L63 (53.35, -31) -> (53.35, -23)
  line L64 (-52.65, -28.75) -> (-52.65, -25.25)
  line L65 (-52.65, -25.25) -> (-52.65, -28.75)
  line L66 (53.35, -28) -> (53.35, -17)
  line L67 (53.35, -17) -> (53.35, -28)
  dimension "d97" = -0.5
  dimension "d98" = 8
  constraint coincident L31.end L32.start
  constraint perpendicular L32 L39
  constraint tangent L39 A0
  constraint vertical L40
  constraint tangent A0 L40
  constraint tangent L38 A1
  constraint coincident L48 A1.end
  constraint coincident L38 A1.end
  constraint tangent L40 A1
  constraint equal A0 A1
  constraint coincident L34.start L37.end
  constraint coincident L30.end L31.start
  constraint horizontal L51
  constraint vertical L52
  constraint horizontal L53
  constraint vertical L54
  constraint coincident L46 L52.end
  constraint coincident L30.start L33.end
  constraint coincident L32.end L52
  constraint horizontal L55
  constraint vertical L56
  constraint horizontal L57
  constraint vertical L58
  constraint coincident L44 L56.end
  constraint coincident L35.end L36.start
  constraint coincident L34.end L56
  constraint symmetric L31.end L59 L36.end
  constraint symmetric L39.end L59 L60.end
  constraint symmetric A0.end L59 A2.start
  constraint symmetric A0 L59 A2
  constraint symmetric A1.end L59 A3.start
  constraint symmetric L40.start L59 L61.start
  constraint symmetric A1 L59 A3
  measures "d98" distance of L40 L46.start
extrude "Extrude19" add sketch "Sketch16" along normal blind 5 separate body contours L30 L31 L32 L33 L51 | L30 L45 L46 L50 L54 L59 | L32 L39 A0 L40 L46 L47 L48 A1 L52 | L34 L44 L45 L50 L56 L59 | L34 L35 L36 L37 L55 | L36 L42 L43 L44 L58 L60 A2 L61 A3 makes body 17
sketch "Sketch17" plane through (-37.85, 0, 0) normal (-1, 0, 0) x (0, -1, 0)
  line L0 (118.6778, -33.485) -> (119.0198, -34.4247)
  line L1 (118.721, -35.0656) -> (115.9019, -36.0916)
  line L2 (115.2611, -35.7928) -> (114.919, -34.8531)
  line L3 (115.2179, -34.2122) -> (118.037, -33.1862)
  line L4 (160.0882, -17.8808) -> (162.9073, -16.8547)
  line L5 (163.5481, -17.1535) -> (163.8902, -18.0932)
  line L6 (163.5913, -18.7341) -> (160.7722, -19.7602)
  line L7 (160.1314, -19.4613) -> (159.7894, -18.5216)
  line L8 (12.7267, -51) -> (12.7267, -58.5)
  line L9 (12.7267, -58.5) -> (59, -58.5)
  arc A0 (59, -58.5) -> (64.1303, -57.5954) centre (59, -43.5) ccw
  line L10 (64.1303, -57.5954) -> (123.9221, -35.8329)
  arc A1 (157.2812, -23.6912) -> (123.9221, -35.8329) centre (140.6017, -29.7621) ccw
  line L11 (157.2812, -23.6912) -> (168.7924, -19.5015)
  arc A2 (168.7924, -19.5015) -> (130.3411, -1.5713) centre (140.6017, -29.7621) ccw
  line L12 (130.3411, -1.5713) -> (79.7087, -20)
  line L13 (79.7087, -20) -> (59, -20)
  line L14 (59, -20) -> (59, -43.5)
  line L15 (59, -43.5) -> (55.5, -43.5)
  line L16 (55.5, -43.5) -> (25.1667, -43.5)
  line L17 (-39, -43.5) -> (-39, -20)
  arc A3 (-39, -20) -> (-54.0001, -35) centre (-39, -35.0001) ccw
  line L18 (-54.0001, -35) -> (-54.0001, -43)
  arc A4 (-54.0001, -43) -> (-38.5465, -58.5) centre (-38.5, -43) ccw
  line L19 (-38.5465, -58.5) -> (7.7267, -58.5)
  line L20 (7.7267, -58.5) -> (7.7267, -51)
  line L21 (7.7267, -51) -> (12.7267, -51)
  arc A5 (157.2812, -23.6912) -> (123.9221, -35.8329) centre (140.6017, -29.7621) ccw
  arc A6 (158.2209, -23.3492) -> (122.9824, -36.175) centre (140.6017, -29.7621) ccw
  line L22 (157.2812, -23.6912) -> (158.0008, -22.7741)
  line L23 (156.8467, -22.6095) -> (158.0008, -22.7741)
  line L24 (156.8467, -22.6095) -> (157.2812, -23.6912)
  arc A7 (160.1314, -19.4613) -> (160.7722, -19.7602) centre (160.6012, -19.2903) ccw
  arc A8 (160.0882, -17.8808) -> (159.7894, -18.5216) centre (160.2592, -18.3506) ccw
  arc A9 (163.5481, -17.1535) -> (162.9073, -16.8547) centre (163.0783, -17.3246) ccw
  arc A10 (163.5913, -18.7341) -> (163.8902, -18.0932) centre (163.4203, -18.2642) ccw
  arc A11 (115.2611, -35.7928) -> (115.9019, -36.0916) centre (115.7309, -35.6218) ccw
  arc A12 (115.2179, -34.2122) -> (114.919, -34.8531) centre (115.3889, -34.6821) ccw
  arc A13 (118.6778, -33.485) -> (118.037, -33.1862) centre (118.208, -33.656) ccw
  arc A14 (118.721, -35.0656) -> (119.0198, -34.4247) centre (118.55, -34.5957) ccw
  line L25 (25.1667, -43.5) -> (-39, -43.5)
  dimension "d101" = 1
  constraint coincident A1.start L11.start
  constraint coincident A6 L22.end
  constraint coincident A5 L23.start
  constraint equal L22 L23
  constraint equal L22 L24
extrude "Extrude20" cut sketch "Sketch17" against normal through all contours A1 A5 L22 L23 | A1 A5 L24 bodies 15 16
pattern_circular "C-Pattern1" count 50 over 180 about axis through (-32.85, -140.6017, -29.7621) along (-1, 0, 0) of "Extrude20"
move_face "OffsetFaces1" offset 0.05 1 faces at (-32.85, -11.0601, -46) on bodies 17
move_face "OffsetFaces2" offset 0.05 1 faces at (32.15, -11.0601, -48.5) on bodies 17
equation "d1 = 79 mm - 0.3 mm"
equation "d2 = 51 mm + 0.3 mm"
equation "d82 = 65 mm + d72 / 2"
equation "d114 = 12 mm + 5 mm"
